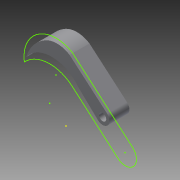
# Autodesk Inventor part: other ratchet piece
Saved by Autodesk Inventor 2013 (Build 170138000, 138)
## iProperties
Created: 2014-01-04
Part Number: other ratchet piece
Material: Generic
Document SubType Name: Modeling
Designer: kahohbein
Density: 1 g/cm^3
Author: kahohbein
Autodesk Inventor part; units mm, degrees
ref_plane "YZ Plane" through (0, 0, 0) normal (1, 0, 0) x (0, 1, 0)
ref_plane "XZ Plane" through (0, 0, 0) normal (0, 1, 0) x (-1, 0, 0)
ref_plane "XY Plane" through (0, 0, 0) normal (0, 0, 1) x (1, 0, 0)
sketch "Sketch1" plane through (0, 0, 0) normal (0, 0, 1) x (1, 0, 0)
  arc A0 (-3.2553, 16.7185) -> (-12.7, 12.6645) centre (-4.6373, 6.9094) ccw
  arc A1 (-6.4227, 20.4471) -> (-12.7, 12.6645) centre (-0.4241, 9.1858) ccw
  arc A2 (1.1505, 20.1734) -> (-6.4227, 20.4471) centre (-2.8721, 13.7815) ccw
  arc A3 (3.9398, 12.6645) -> (-3.2553, 16.7185) centre (-4.2623, 6.5193) ccw
  line L0 (1.1505, 20.1734) -> (13.1197, 9.9539)
  line L1 (3.9398, 12.6645) -> (10.1839, 6.7025)
  arc A4 (10.1837, 6.7027) -> (13.1197, 9.9539) centre (11.6969, 8.2875) ccw
  point P0 (0, 0)
  point P1 (-12.7, 0)
  dimension "d0" = 9.906
  constraints: 10 point on circle, 5 centre point, 4 end point, 3 tangent, 1 point on line
  measures "d0" radius of A0
extrude "Extrusion1" add sketch "Sketch1" along normal blind 6.35
sketch "Sketch2" plane through (0, 0, 6.35) normal (0, 0, 1) x (1, 0, 0)
  arc A0 (10.1837, 6.7027) -> (13.1197, 9.9539) centre (11.6969, 8.2875) ccw projected
  circle A1 centre (11.6969, 8.2875) radius 1.143
  point P0 (0, 0)
  dimension "d3" = 2.286
  constraints: 1 centre point, 1 coincident
  measures "d3" diameter of A1
extrude "Extrusion2" cut sketch "Sketch2" against normal blind 25.4
sketch "Sketch3" plane through (0, 0, 6.35) normal (0, 0, 1) x (1, 0, 0)
  arc A0 (16.5583, -0.6886) -> (21.2023, 4.6943) centre (18.8803, 2.0028) ccw
  line L0 (21.2023, 4.6943) -> (1.9212, 21.3289)
  line L1 (16.5583, -0.6886) -> (1.9487, 11.9157)
  arc A1 (1.9487, 11.9157) -> (-13.3635, 11.0028) centre (-5.238, 3.5857) ccw
  arc A2 (1.9212, 21.3289) -> (-13.3635, 11.0028) centre (-3.1996, 12.4333) ccw
  point P0 (0, 0)
  constraints: 6 point on circle, 4 end point, 3 centre point, 3 tangent, 1 parallel
body "Solid1"
